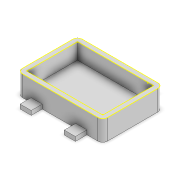
# Autodesk Inventor part: Gyro_box_bottom
Saved by Autodesk Inventor 2020 (Build 240168000, 168)
## iProperties
Created: 2019-08-08
Part Number: Gyro_box_bottom
Material: Generic
Document SubType Name: Modeling
Designer: chitl
Density: 1 g/cm^3
Appearance: Default
Author: chitl
Autodesk Inventor part; units mm, degrees
ref_plane "YZ Plane" through (0, 0, 0) normal (1, 0, 0) x (0, 1, 0)
ref_plane "XZ Plane" through (0, 0, 0) normal (0, 1, 0) x (-1, 0, 0)
sketch "Sketch1" plane through (0, 0, 0) normal (0, 1, 0) x (-1, 0, 0)
  line L0 (-2.922, 0) -> (47.078, 0)
  line L1 (47.078, 0) -> (47.078, 33.0962)
  line L2 (47.078, 33.0962) -> (-2.922, 33.0962)
  line L3 (-2.922, 33.0962) -> (-2.922, 0)
  line L4 (50.578, 36.5962) -> (50.578, -3.5)
  line L5 (50.578, -3.5) -> (-6.422, -3.5)
  line L6 (-6.422, -3.5) -> (-6.422, 36.5962)
  line L7 (-6.422, 36.5962) -> (50.578, 36.5962)
  point P0 (0, 0)
  dimension "d0" = 50
  dimension "d1" = 33.0962
  dimension "d2" = 3.5
  constraints: 16 end point, 4 parallel, 2 perpendicular, 1 horizontal, 3 other
  measures "d0" distance of L2.end L1.end
  measures "d1" distance of L1.end L0.end
  measures "d2" distance between parallel lines of L1 L4
extrude "Extrusion1" add sketch "Sketch1" along normal blind 13.97 contours L3 L2 L1 L0 | L4 L5 L6 L7
shell "Shell1" thickness 3 removed faces 0
sketch "Sketch2" plane through (0, 13.97, 0) normal (0, 1, 0) x (1, 0, 0)
  point P0 (0, 0)
move faces "Move1" translate (0, -3.175, 0) faces at (-12.578, 13.97, 23.2308)
move faces "Move2" translate (0, 3, 0) faces at (-13.578, 10.795, 35.5962)
fillet "Fillet1" radius 3.175 4 edges at (6.422, 6.8975, 36.5962) (6.422, 6.8975, -3.5) (-50.578, 6.8975, -3.5) (-50.578, 6.8975, 36.5962)
ref_plane "Work Plane1" through (-47.403, 13.795, 36.5962) normal (0, 1, 0) x (1, 0, 0)
sketch "Sketch3" plane through (-47.403, 13.795, 36.5962) normal (0, 1, 0) x (1, 0, 0)
  arc A0 (-3.175, 3.175) -> (0, 0) centre (0, 3.175) ccw projected
  line L0 (0, 0) -> (50.65, 0) projected
  arc A1 (50.65, 0) -> (53.825, 3.175) centre (50.65, 3.175) ccw projected
  line L1 (53.825, 3.175) -> (53.825, 36.9212) projected
  arc A2 (53.825, 36.9212) -> (50.65, 40.0962) centre (50.65, 36.9212) ccw projected
  line L2 (50.65, 40.0962) -> (0, 40.0962) projected
  arc A3 (0, 40.0962) -> (-3.175, 36.9212) centre (0, 36.9212) ccw projected
  line L3 (-3.175, 36.9212) -> (-3.175, 3.175) projected
  line L4 (50.825, 3) -> (-0.175, 3) projected
  line L5 (-0.175, 3) -> (-0.175, 37.0962) projected
  line L6 (-0.175, 37.0962) -> (50.825, 37.0962) projected
  line L7 (50.825, 37.0962) -> (50.825, 3) projected
  point P0 (47.403, 36.5962)
sketch "Sketch4" plane through (0, 0, 0) normal (0, -1, 0) x (1, 0, 0)
  arc A0 (-50.578, 33.4212) -> (-47.403, 36.5962) centre (-47.403, 33.4212) ccw projected
  line L0 (-50.578, -0.325) -> (-50.578, 33.4212) projected
  arc A1 (-47.403, -3.5) -> (-50.578, -0.325) centre (-47.403, -0.325) ccw projected
  line L1 (3.247, -3.5) -> (-47.403, -3.5)
  arc A2 (6.422, -0.325) -> (3.247, -3.5) centre (3.247, -0.325) ccw projected
  line L2 (6.422, 33.4212) -> (6.422, -0.325) projected
  arc A3 (3.247, 36.5962) -> (6.422, 33.4212) centre (3.247, 33.4212) ccw projected
  line L3 (-47.403, 36.5962) -> (3.247, 36.5962)
  line L4 (-41.4583, 43.9872) -> (-33.9992, 43.9872)
  line L5 (-33.9992, 43.9872) -> (-33.9992, -11.1575)
  line L6 (-33.9992, -11.1575) -> (-41.4583, -11.1575)
  line L7 (-41.4583, -11.1575) -> (-41.4583, 43.9872)
  line L8 (-11.5895, 44.289) -> (-4.1219, 44.289)
  line L9 (-4.1219, 44.289) -> (-4.1219, -11.1575)
  line L10 (-4.1219, -11.1575) -> (-11.5895, -11.1575)
  line L11 (-11.5895, -11.1575) -> (-11.5895, 44.289)
  point P0 (0, 0)
  dimension "d15" = 7.4591
  dimension "d16" = 55.1447
  dimension "d17" = 7.4676
  constraints: 20 end point, 4 centre point, 4 parallel, 2 horizontal, 2 perpendicular
  measures "d15" distance of L5.end L6.end
  measures "d16" distance of L4.end L5.end
  measures "d17" distance of L9.end L10.end
extrude "Extrusion2" add sketch "Sketch4" against normal blind 2.8575 contours L7 L4 L5 L3 | L3 L5 L1 L7 | L1 L5 L6 L7 | L11 L8 L9 L3 | L3 L9 L1 L11 | L1 L9 L10 L11
body "Solid1"
